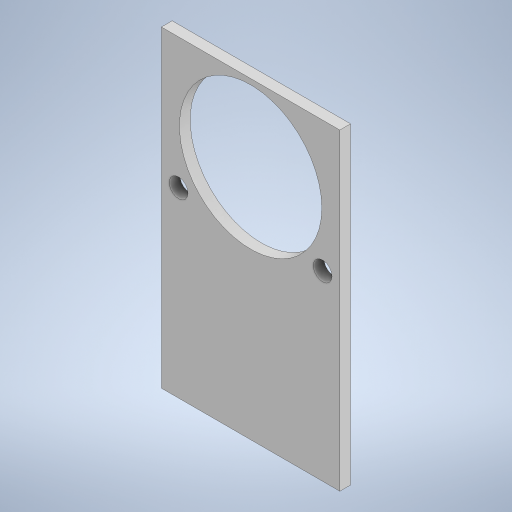
# Autodesk Inventor part: Motor_Cover
Saved by Autodesk Inventor 2023.5 (Build 275446020, 446B)
## iProperties
Created: 2025-04-14
Part Number: Motor_Cover
Material: Generic
Document SubType Name: Modeling
Designer: Lucky Sah
Density: 1 g/cm^3
Appearance: Default
Author: Lucky Sah
Autodesk Inventor part; units mm, degrees
ref_plane "YZ Plane" through (0, 0, 0) normal (1, 0, 0) x (0, 1, 0)
ref_plane "XZ Plane" through (0, 0, 0) normal (0, 1, 0) x (-1, 0, 0)
ref_plane "XY Plane" through (0, 0, 0) normal (0, 0, 1) x (1, 0, 0)
sketch "Sketch1" plane through (0, 0, 0) normal (0, 0, 1) x (1, 0, 0)
  line L0 (-58.7621, -16.3299) -> (-25.5621, -16.3299)
  line L1 (-25.5621, -16.3299) -> (-25.5621, 41.8701)
  line L2 (-25.5621, 41.8701) -> (-58.7621, 41.8701)
  line L3 (-58.7621, 41.8701) -> (-58.7621, -16.3299)
  line L4 (-66.7621, 49.8701) -> (-17.5621, 49.8701)
  line L5 (-17.5621, 49.8701) -> (-17.5621, -24.3299)
  line L6 (-17.5621, -24.3299) -> (-66.7621, -24.3299)
  line L7 (-66.7621, -24.3299) -> (-66.7621, 49.8701)
  line L8 (-2.5621, -24.3299) -> (-2.5621, 49.8701)
  line L9 (-17.5621, 64.8701) -> (-66.7621, 64.8701)
  line L10 (-81.7621, 49.8701) -> (-81.7621, -24.3299)
  line L11 (-66.7621, -39.3299) -> (-17.5621, -39.3299)
  circle A0 centre (-10.0621, 45.8701) radius 2.55
  circle A1 centre (-10.0621, -20.3299) radius 2.55
  circle A2 centre (-74.2621, 45.8701) radius 2.55
  circle A3 centre (-74.2621, -20.3299) radius 2.55
  arc A4 (-66.7621, 64.8701) -> (-81.7621, 49.8701) centre (-66.7621, 49.8701) ccw
  arc A5 (-2.5621, 49.8701) -> (-17.5621, 64.8701) centre (-17.5621, 49.8701) ccw
  arc A6 (-17.5621, -39.3299) -> (-2.5621, -24.3299) centre (-17.5621, -24.3299) ccw
  arc A7 (-81.7621, -24.3299) -> (-66.7621, -39.3299) centre (-66.7621, -24.3299) ccw
  circle A8 centre (-42.1621, 27.6201) radius 13.25
  circle A9 centre (-55.5621, 17.5701) radius 1.75
  circle A10 centre (-28.7621, 17.5701) radius 1.75
  point P0 (0, 0)
  dimension "d0" = 58.2
  dimension "d1" = 33.2
  dimension "d2" = 8
  dimension "d3" = 15
  dimension "d4" = 5.1
  dimension "d5" = 7.5
  dimension "d6" = 5.1
  dimension "d7" = 5.1
  dimension "d8" = 7.5
  dimension "d9" = 5.1
  dimension "d10" = 4
  dimension "d11" = 4
  dimension "d12" = 4
  dimension "d13" = 4
  dimension "d14" = 7.5
  dimension "d15" = 7.5
  dimension "d16" = 15
  dimension "d17" = 26.5
  dimension "d18" = 14.25
  dimension "d19" = 3.5
  dimension "d20" = 24.3
  dimension "d21" = 3.2
  dimension "d22" = 3.5
  dimension "d23" = 24.3
  dimension "d24" = 3.2
  constraints: 24 end point, 11 centre point, 8 point on circle, 8 tangent, 6 parallel, 3 equal radius, 3 perpendicular, 1 horizontal, 6 other
  measures "d0" distance between parallel lines of L0 L2
  measures "d1" distance between parallel lines of L1 L3
  measures "d2" distance between parallel lines of L2 L4
  measures "d3" distance between parallel lines of L5 L8
  measures "d4" diameter of A0
  measures "d5" distance from line of L5 A0.centre
  measures "d6" diameter of A1
  measures "d7" diameter of A2
  measures "d8" distance from line of L7 A2.centre
  measures "d9" diameter of A3
  measures "d10" distance from line of L4 A0.centre
  measures "d11" distance from line of L6 A1.centre
  measures "d12" distance from line of L4 A2.centre
  measures "d13" distance from line of L6 A3.centre
  measures "d14" distance from line of L7 A3.centre
  measures "d15" distance from line of L8 A1.centre
  measures "d16" radius of A4
  measures "d17" diameter of A8
  measures "d18" distance from line of A8.centre L2
  measures "d19" diameter of A9
  measures "d20" distance from line of A9.centre L2
  measures "d21" distance from line of L3 A9.centre
  measures "d22" diameter of A10
  measures "d23" distance from line of A10.centre L2
  measures "d24" distance from line of L1 A10.centre
extrude "Extrusion1" add sketch "Sketch1" along normal blind 2 contours L3 L2 L1 L0
body "Solid1"
